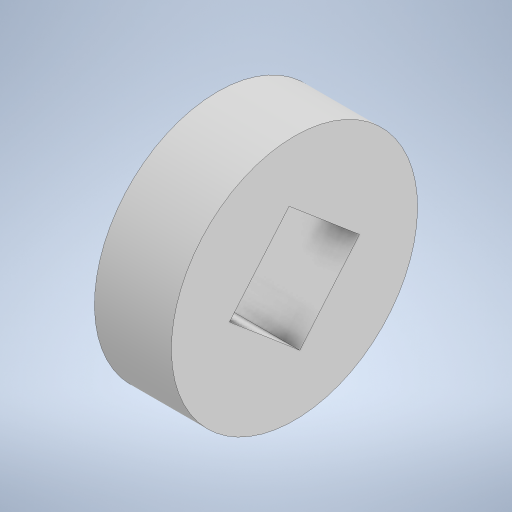
# Autodesk Inventor part: Задание номер 7
Saved by Autodesk Inventor 2023.2 (Build 272271030, 271C)
## iProperties
Created: 2023-09-07
Part Number: Задание номер 7
Material: Типовые
Document SubType Name: Modeling
Designer: User
Density: 1 g/cm^3
Appearance: По умолчанию
Author: User
Autodesk Inventor part; units mm, degrees
ref_plane "YZ Plane" through (0, 0, 0) normal (1, 0, 0) x (0, 1, 0)
ref_plane "XZ Plane" through (0, 0, 0) normal (0, 1, 0) x (-1, 0, 0)
ref_plane "XY Plane" through (0, 0, 0) normal (0, 0, 1) x (1, 0, 0)
sketch "Эскиз1" plane through (0, 0, 0) normal (1, 0, 0) x (0, 1, 0)
  circle A0 centre (13.1151, 9.6132) radius 16
  line L0 (12.4181, 18.0698) -> (21.5717, 10.3101)
  line L1 (21.5717, 10.3101) -> (13.812, 1.1566)
  line L2 (13.812, 1.1566) -> (4.6584, 8.9163)
  line L3 (4.6584, 8.9163) -> (12.4181, 18.0698)
  line L4 (12.4181, 18.0698) -> (13.812, 1.1566) construction
  point P0 (0, 0)
  dimension "d0" = 32
  dimension "d2" = 12
  constraints: 10 end point, 2 parallel, 1 centre point, 1 midpoint, 1 perpendicular
  measures "d0" diameter of A0
  measures "d2" distance of L0.end L1.end
extrude "Выдавливание1" add sketch "Эскиз1" along normal blind 10
